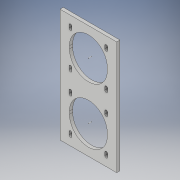
# Autodesk Inventor part: z gearing adapter
Saved by Autodesk Inventor 2019 (Build 230136000, 136)
## iProperties
Created: 2018-07-27
Part Number: z gearing adapter
Material: Generic
Document SubType Name: Modeling
Designer: torba
Density: 1 g/cm^3
Appearance: Default
Author: torba
Autodesk Inventor part; units mm, degrees
ref_plane "YZ Plane" through (0, 0, 0) normal (1, 0, 0) x (0, 1, 0)
ref_plane "XZ Plane" through (0, 0, 0) normal (0, 1, 0) x (-1, 0, 0)
ref_plane "XY Plane" through (0, 0, 0) normal (0, 0, 1) x (1, 0, 0)
sketch "Sketch1" plane through (0, 0, 0) normal (0, 0, 1) x (1, 0, 0)
  arc A0 (44.2015, -79.5823) -> (38.6015, -79.5823) centre (41.4015, -79.5823) ccw
  arc A1 (38.6015, -85.1823) -> (44.2015, -85.1823) centre (41.4015, -85.1823) ccw
  line L0 (38.6015, -85.1823) -> (38.6015, -79.5823)
  line L1 (44.2015, -79.5823) -> (44.2015, -85.1823)
  arc A2 (39.4335, -50.3778) -> (112.9665, -50.3778) centre (76.2, -50.3778) ccw
  arc A3 (112.9665, -44.7898) -> (39.4335, -44.7898) centre (76.2, -44.7898) ccw
  line L2 (39.4335, -50.3778) -> (39.4335, -44.7898)
  line L3 (112.9665, -44.7898) -> (112.9665, -50.3778)
  line L4 (44.2015, -9.9853) -> (44.2015, -15.5853)
  arc A4 (44.2015, -9.9853) -> (38.6015, -9.9853) centre (41.4015, -9.9853) ccw
  line L5 (38.6015, -15.5853) -> (38.6015, -9.9853)
  arc A5 (38.6015, -15.5853) -> (44.2015, -15.5853) centre (41.4015, -15.5853) ccw
  line L6 (108.1985, -85.1823) -> (108.1985, -79.5823)
  arc A6 (108.1985, -85.1823) -> (113.7985, -85.1823) centre (110.9985, -85.1823) ccw
  line L7 (113.7985, -79.5823) -> (113.7985, -85.1823)
  arc A7 (113.7985, -79.5823) -> (108.1985, -79.5823) centre (110.9985, -79.5823) ccw
  line L8 (108.1985, -15.5853) -> (108.1985, -9.9853)
  arc A8 (113.7985, -9.9853) -> (108.1985, -9.9853) centre (110.9985, -9.9853) ccw
  line L9 (113.7985, -9.9853) -> (113.7985, -15.5853)
  arc A9 (108.1985, -15.5853) -> (113.7985, -15.5853) centre (110.9985, -15.5853) ccw
  circle A10 centre (76.2, -47.5838) radius 1.27
  line L10 (6.35, 0.0014) -> (6.35, -109.7489)
  line L11 (152.4, 0) -> (0, 0)
  line L12 (146.05, 0.0027) -> (146.05, -109.7476)
  line L13 (0, -109.7503) -> (152.4, -109.7503)
  line L14 (21.2, 7.4162) -> (131.2, 7.4162)
  line L15 (131.2, 7.4162) -> (131.2, -102.5838)
  line L16 (131.2, -102.5838) -> (21.2, -102.5838)
  line L17 (21.2, -102.5838) -> (21.2, 7.4162)
  line L18 (21.2, 7.4162) -> (131.2, -102.5838) construction
  line L19 (131.2, 7.4162) -> (21.2, -102.5838) construction
  dimension "d0" = 2.8
  dimension "d1" = 36.7665
  dimension "d2" = 2.54
  dimension "d3" = 90
  dimension "d4" = 90
  dimension "d5" = 90
  dimension "d6" = 90
  dimension "d7" = 109.7503
  dimension "d8" = 32.2515
  dimension "d9" = 33.0835
  dimension "d10" = 101.8485
  dimension "d11" = 139.7
  dimension "d12" = 6.35
  dimension "d13" = 38.6015
  dimension "d14" = 6.35
  dimension "d15" = 0.0027
  dimension "d16" = 37.8515
  dimension "d17" = 109.7476
  dimension "d18" = 9.9853
  dimension "d19" = 69.597
  dimension "d20" = 75.197
  dimension "d21" = 79.5823
  dimension "d22" = 44.7898
  dimension "d23" = 50.3778
  dimension "d24" = 47.5838
  dimension "d25" = 69.85
  dimension "d26" = 9.9853
  dimension "d27" = 79.5823
  dimension "d28" = 0.0014
  dimension "d29" = 109.7489
  dimension "d30" = 146.05
  dimension "d31" = 146.05
  dimension "d32" = 110
  dimension "d33" = 110
  dimension "d34" = 17.4015
  constraints: 40 end point, 24 tangent, 20 point on circle, 11 centre point, 10 parallel, 2 horizontal, 2 midpoint, 1 equal radius, 1 perpendicular, 1 vertical
  measures "d0" radius of A8
  measures "d1" radius of A3
  measures "d2" diameter of A10
  measures "d3" angle of L11 L9
  measures "d4" angle of L11 L8
  measures "d5" angle of L11 L1
  measures "d6" angle of L11 L0
  measures "d7" distance between parallel lines of L11 L13
  measures "d8" distance between parallel lines of L12 L7
  measures "d9" distance between parallel lines of L12 L3
  measures "d10" distance between parallel lines of L12 L4
  measures "d11" distance between parallel lines of L12 L10
  measures "d12" distance from line of L11.start L12
  measures "d13" distance from line of L11.start L9
  measures "d14" distance from line of L13.end L12
  measures "d15" distance from line of L12.start L11
  measures "d16" distance from line of L12.start L8
  measures "d17" distance from line of L12.end L11
  measures "d18" distance from line of L9.start L11
  measures "d19" distance from line of L9.start L1
  measures "d20" distance from line of L9.start L0
  measures "d21" distance from line of L7.start L11
  measures "d22" distance from line of L3.start L11
  measures "d23" distance from line of L3.end L11
  measures "d24" distance from line of A10.centre L11
  measures "d25" distance from line of A10.centre L12
  measures "d26" distance from line of L4.start L11
  measures "d27" distance from line of L1.start L11
  measures "d28" distance from line of L10.start L11
  measures "d29" distance from line of L10.end L11
  measures "d30" distance from line of L11.end L12
  measures "d31" distance from line of L13.start L12
  measures "d32" distance between parallel lines of L15 L17
  measures "d33" distance between parallel lines of L16 L14
  measures "d34" distance from line of L16 A1.centre
extrude "Extrusion1" add sketch "Sketch1" along normal blind 6.35 contours L15 L16 L17 L11 | L11 L17 L14 L15
sketch "Sketch3" plane through (0, 0, 6.35) normal (0, 0, 1) x (1, 0, 0)
  line L0 (112.9665, -44.7898) -> (112.9665, -50.3778) projected
  arc A0 (39.4335, -50.3778) -> (112.9665, -50.3778) centre (76.2, -50.3778) ccw projected
  line L1 (39.4335, -50.3778) -> (39.4335, -44.7898) projected
  arc A1 (112.9665, -44.7898) -> (39.4335, -44.7898) centre (76.2, -44.7898) ccw projected
  arc A2 (38.6015, -15.5853) -> (44.2015, -15.5853) centre (41.4015, -15.5853) ccw projected
  line L2 (38.6015, -15.5853) -> (38.6015, -9.9853) projected
  arc A3 (44.2015, -9.9853) -> (38.6015, -9.9853) centre (41.4015, -9.9853) ccw projected
  line L3 (44.2015, -9.9853) -> (44.2015, -15.5853) projected
  line L4 (44.2015, -79.5823) -> (44.2015, -85.1823) projected
  arc A4 (38.6015, -85.1823) -> (44.2015, -85.1823) centre (41.4015, -85.1823) ccw projected
  line L5 (38.6015, -85.1823) -> (38.6015, -79.5823) projected
  arc A5 (44.2015, -79.5823) -> (38.6015, -79.5823) centre (41.4015, -79.5823) ccw projected
  arc A6 (113.7985, -79.5823) -> (108.1985, -79.5823) centre (110.9985, -79.5823) ccw projected
  line L6 (113.7985, -79.5823) -> (113.7985, -85.1823) projected
  arc A7 (108.1985, -85.1823) -> (113.7985, -85.1823) centre (110.9985, -85.1823) ccw projected
  line L7 (108.1985, -85.1823) -> (108.1985, -79.5823) projected
  arc A8 (113.7985, -9.9853) -> (108.1985, -9.9853) centre (110.9985, -9.9853) ccw projected
  line L8 (113.7985, -9.9853) -> (113.7985, -15.5853) projected
  arc A9 (108.1985, -15.5853) -> (113.7985, -15.5853) centre (110.9985, -15.5853) ccw projected
  line L9 (108.1985, -15.5853) -> (108.1985, -9.9853) projected
  line L10 (131.2, 7.4162) -> (21.2, 7.4162) projected
  line L11 (21.2, 7.4162) -> (21.2, -102.5838) projected
  line L12 (21.2, -102.5838) -> (131.2, -102.5838) projected
  line L13 (131.2, -102.5838) -> (131.2, 7.4162) projected
  line L14 (112.9665, 65.2102) -> (112.9665, 59.6222)
  arc A10 (39.4335, 59.6222) -> (112.9665, 59.6222) centre (76.2, 59.6222) ccw
  line L15 (39.4335, 59.6222) -> (39.4335, 65.2102)
  arc A11 (112.9665, 65.2102) -> (39.4335, 65.2102) centre (76.2, 65.2102) ccw
  arc A12 (38.6015, 94.4147) -> (44.2015, 94.4147) centre (41.4015, 94.4147) ccw
  line L16 (38.6015, 94.4147) -> (38.6015, 100.0147)
  arc A13 (44.2015, 100.0147) -> (38.6015, 100.0147) centre (41.4015, 100.0147) ccw
  line L17 (44.2015, 100.0147) -> (44.2015, 94.4147)
  line L18 (44.2015, 30.4177) -> (44.2015, 24.8177)
  arc A14 (38.6015, 24.8177) -> (44.2015, 24.8177) centre (41.4015, 24.8177) ccw
  line L19 (38.6015, 24.8177) -> (38.6015, 30.4177)
  arc A15 (44.2015, 30.4177) -> (38.6015, 30.4177) centre (41.4015, 30.4177) ccw
  arc A16 (113.7985, 30.4177) -> (108.1985, 30.4177) centre (110.9985, 30.4177) ccw
  line L20 (113.7985, 30.4177) -> (113.7985, 24.8177)
  arc A17 (108.1985, 24.8177) -> (113.7985, 24.8177) centre (110.9985, 24.8177) ccw
  line L21 (108.1985, 24.8177) -> (108.1985, 30.4177)
  arc A18 (113.7985, 100.0147) -> (108.1985, 100.0147) centre (110.9985, 100.0147) ccw
  line L22 (113.7985, 100.0147) -> (113.7985, 94.4147)
  arc A19 (108.1985, 94.4147) -> (113.7985, 94.4147) centre (110.9985, 94.4147) ccw
  line L23 (108.1985, 94.4147) -> (108.1985, 100.0147)
  line L24 (131.2, 117.4162) -> (21.2, 117.4162)
  line L25 (21.2, 117.4162) -> (21.2, 7.4162)
  line L26 (21.2, 7.4162) -> (131.2, 7.4162)
  line L27 (131.2, 7.4162) -> (131.2, 117.4162)
  point P0 (0, 0)
  dimension "d37" = 90
  dimension "d38" = 90
  dimension "d39" = 90
  dimension "d40" = 90
  dimension "d41" = 90
  dimension "d42" = 90
  dimension "d43" = 90
  dimension "d44" = 90
  dimension "d45" = 90
  dimension "d46" = 90
  dimension "d47" = 90
  dimension "d48" = 90
  dimension "d49" = 90
  dimension "d50" = 110
  dimension "d51" = 0
  dimension "d52" = 17.4015
  dimension "d53" = 17.4015
  dimension "d54" = 18.2335
  dimension "d55" = 23.0015
  dimension "d56" = 23.0015
  dimension "d57" = 86.9985
  dimension "d58" = 86.9985
  dimension "d59" = 91.7665
  dimension "d60" = 92.5985
  dimension "d61" = 92.5985
  dimension "d62" = 110
  dimension "d63" = 0
  dimension "d64" = 92.5985
  dimension "d65" = 23.0015
  dimension "d66" = 57.794
  dimension "d67" = 52.206
  dimension "d68" = 92.5985
  dimension "d69" = 23.0015
  constraints: 28 end point, 24 tangent, 20 point on circle, 10 centre point, 1 parallel
  measures "d37" angle of L10 L27
  measures "d38" angle of L10 L22
  measures "d39" angle of L10 L20
  measures "d40" angle of L10 L14
  measures "d41" angle of L10 L23
  measures "d42" angle of L10 L21
  measures "d43" angle of L10 L17
  measures "d44" angle of L10 L18
  measures "d45" angle of L10 L15
  measures "d46" angle of L10 L16
  measures "d47" angle of L10 L19
  measures "d48" angle of L10 L25
  measures "d49" angle of L13 L26
  measures "d50" distance between parallel lines of L10 L24
  measures "d51" distance from line of L10.start L27
  measures "d52" distance from line of L10.start L22
  measures "d53" distance from line of L10.start L20
  measures "d54" distance from line of L10.start L14
  measures "d55" distance from line of L10.start L23
  measures "d56" distance from line of L10.start L21
  measures "d57" distance from line of L10.start L17
  measures "d58" distance from line of L10.start L18
  measures "d59" distance from line of L10.start L15
  measures "d60" distance from line of L10.start L16
  measures "d61" distance from line of L10.start L19
  measures "d62" distance from line of L10.start L25
  measures "d63" distance from line of L10.start L26
  measures "d64" distance from line of L22.start L10
  measures "d65" distance from line of L20.start L10
  measures "d66" distance from line of L14.start L10
  measures "d67" distance from line of L14.end L10
  measures "d68" distance from line of L17.start L10
  measures "d69" distance from line of L18.start L10
extrude "Extrusion2" add sketch "Sketch3" against normal blind 6.35 contours L10 L25 L24 L27
sketch "Sketch4" plane through (0, 0, 6.35) normal (0, 0, 1) x (1, 0, 0)
  arc A0 (44.2015, 30.4177) -> (38.6015, 30.4177) centre (41.4015, 30.4177) ccw projected
  line L0 (44.2015, 30.4177) -> (44.2015, 24.8177) projected
  arc A1 (38.6015, 24.8177) -> (44.2015, 24.8177) centre (41.4015, 24.8177) ccw projected
  line L1 (38.6015, 24.8177) -> (38.6015, 30.4177) projected
  line L2 (113.7985, 100.0147) -> (113.7985, 94.4147) projected
  arc A2 (108.1985, 94.4147) -> (113.7985, 94.4147) centre (110.9985, 94.4147) ccw projected
  line L3 (108.1985, 94.4147) -> (108.1985, 100.0147) projected
  arc A3 (113.7985, 100.0147) -> (108.1985, 100.0147) centre (110.9985, 100.0147) ccw projected
  line L4 (44.2015, 100.0147) -> (44.2015, 94.4147) projected
  arc A4 (38.6015, 94.4147) -> (44.2015, 94.4147) centre (41.4015, 94.4147) ccw projected
  line L5 (38.6015, 94.4147) -> (38.6015, 100.0147) projected
  arc A5 (44.2015, 100.0147) -> (38.6015, 100.0147) centre (41.4015, 100.0147) ccw projected
  line L6 (108.1985, 24.8177) -> (108.1985, 30.4177) projected
  arc A6 (113.7985, 30.4177) -> (108.1985, 30.4177) centre (110.9985, 30.4177) ccw projected
  line L7 (113.7985, 30.4177) -> (113.7985, 24.8177) projected
  arc A7 (108.1985, 24.8177) -> (113.7985, 24.8177) centre (110.9985, 24.8177) ccw projected
  arc A8 (112.9665, 65.2102) -> (39.4335, 65.2102) centre (76.2, 65.2102) ccw projected
  line L8 (112.9665, 65.2102) -> (112.9665, 59.6222) projected
  arc A9 (39.4335, 59.6222) -> (112.9665, 59.6222) centre (76.2, 59.6222) ccw projected
  line L9 (39.4335, 59.6222) -> (39.4335, 65.2102) projected
  line L10 (112.9665, -44.7898) -> (112.9665, -50.3778) projected
  arc A10 (39.4335, -50.3778) -> (112.9665, -50.3778) centre (76.2, -50.3778) ccw projected
  line L11 (39.4335, -50.3778) -> (39.4335, -44.7898) projected
  arc A11 (112.9665, -44.7898) -> (39.4335, -44.7898) centre (76.2, -44.7898) ccw projected
  arc A12 (38.6015, -15.5853) -> (44.2015, -15.5853) centre (41.4015, -15.5853) ccw projected
  line L12 (38.6015, -15.5853) -> (38.6015, -9.9853) projected
  arc A13 (44.2015, -9.9853) -> (38.6015, -9.9853) centre (41.4015, -9.9853) ccw projected
  line L13 (44.2015, -9.9853) -> (44.2015, -15.5853) projected
  line L14 (44.2015, -79.5823) -> (44.2015, -85.1823) projected
  arc A14 (38.6015, -85.1823) -> (44.2015, -85.1823) centre (41.4015, -85.1823) ccw projected
  line L15 (38.6015, -85.1823) -> (38.6015, -79.5823) projected
  arc A15 (44.2015, -79.5823) -> (38.6015, -79.5823) centre (41.4015, -79.5823) ccw projected
  arc A16 (113.7985, -79.5823) -> (108.1985, -79.5823) centre (110.9985, -79.5823) ccw projected
  line L16 (113.7985, -79.5823) -> (113.7985, -85.1823) projected
  arc A17 (108.1985, -85.1823) -> (113.7985, -85.1823) centre (110.9985, -85.1823) ccw projected
  line L17 (108.1985, -85.1823) -> (108.1985, -79.5823) projected
  arc A18 (113.7985, -9.9853) -> (108.1985, -9.9853) centre (110.9985, -9.9853) ccw projected
  line L18 (113.7985, -9.9853) -> (113.7985, -15.5853) projected
  arc A19 (108.1985, -15.5853) -> (113.7985, -15.5853) centre (110.9985, -15.5853) ccw projected
  line L19 (108.1985, -15.5853) -> (108.1985, -9.9853) projected
  line L20 (21.2, -102.5838) -> (21.2, 117.4162) projected
  line L21 (21.2, -102.5838) -> (131.2, -102.5838) projected
  line L22 (131.2, -102.5838) -> (131.2, 117.4162) projected
  line L23 (21.2, 117.4162) -> (131.2, 117.4162) projected
  line L24 (76.2, -50.3778) -> (76.2, -44.7898)
  line L25 (76.2, 59.6222) -> (76.2, 65.2102)
  circle A20 centre (76.2, -47.5838) radius 0.5
  circle A21 centre (76.2, 62.4162) radius 0.5
  point P0 (0, 0)
  dimension "d72" = 1
  dimension "d73" = 1
  constraints: 4 end point, 2 centre point, 2 midpoint, 2 vertical
  measures "d72" diameter of A20
  measures "d73" diameter of A21
extrude "Extrusion3" add sketch "Sketch4" against normal blind 6.35 contours A20 L24 | L24 A20 | A21 L25 | L25 A21
body "Solid1"
